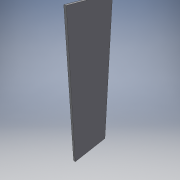
# Autodesk Inventor part: back board (for assembly)
Saved by Autodesk Inventor 2016 (Build 200138000, 138)
## iProperties
Created: 2017-10-23
Part Number: back board (for assembly)
Material: Generic
Document SubType Name: Modeling
Designer: student
Density: 1 g/cm^3
Appearance: Default
Author: student
Autodesk Inventor part; units mm, degrees
ref_plane "YZ Plane" through (0, 0, 0) normal (1, 0, 0) x (0, 1, 0)
ref_plane "XZ Plane" through (0, 0, 0) normal (0, 1, 0) x (-1, 0, 0)
ref_plane "XY Plane" through (0, 0, 0) normal (0, 0, 1) x (1, 0, 0)
sketch "Sketch1" plane through (0, 0, 0) normal (1, 0, 0) x (0, 1, 0)
  line L0 (-787.4, -228.6) -> (787.4, -228.6)
  line L1 (787.4, -228.6) -> (787.4, 228.6)
  line L2 (787.4, 228.6) -> (-787.4, 228.6)
  line L3 (-787.4, 228.6) -> (-787.4, -228.6)
  line L4 (-787.4, -228.6) -> (787.4, 228.6) construction
  line L5 (787.4, -228.6) -> (-787.4, 228.6) construction
  point P0 (0, 0)
  dimension "d0" = 1574.8
  dimension "d1" = 457.2
  constraints: 12 end point, 2 midpoint, 2 parallel, 1 horizontal, 1 perpendicular
  measures "d0" distance of L1.end L2.end
  measures "d1" distance of L0.end L1.end
extrude "Extrusion1" add sketch "Sketch1" along normal blind 25.4
body "Solid1"
